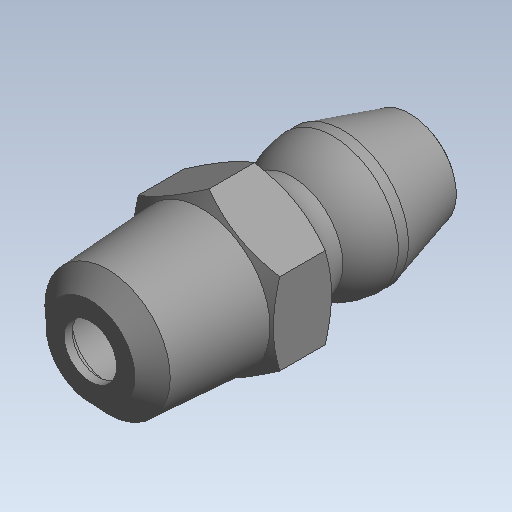
# Autodesk Inventor part: 1/4-28 SAE-LT
Saved by Autodesk Inventor 2020 (Build 240168000, 168)
## iProperties
Part Number: 1/4-28 SAE-LT
Material: Generic
Catalog Web Link: www.cadenas.de
Description: 1/4-28 SAE-LT-Grease Nipple
Vendor: SKF
Document SubType Name: Modeling
Designer: partserver
Manufacturer: SKF
Mass: 0.360827 g
Surface Area: 5.48785 cm^2
Volume: 0.360827 cm^3
Density: 1 g/cm^3
Appearance: PSOLRGB-175-175-175
Category: PARTsolutions
Company: SKF
PSOL_IDENT_0: {$CADENAS_DATA\23d-libs\skf\bearings_units_and_housings\bearing_units\ball_bearing_units\y-unit_acce
PSOL_IDENT_1: ssories\grease_nipple.prj},173 {VTYP=3D},{NB=1/4-28 SAE-LT},{LINA=1/4-28 SAE-LT},{NN=1/4-28 SAE-LT},
PSOL_IDENT_2: {DATE=20.08.2020 13:45:09},{GEOMDATE=29.07.2020 11:16:44},{VERSION=},{LINEID=10},{WBVAR=},{WBNUMERIC=
PSOL_IDENT_3: }  {NB=1/4-28 SAE-LT},{LINA=1/4-28 SAE-LT},{KT=DUMMY},{PN=1/4-28 SAE-LT}
NB: 1/4-28 SAE-LT
NN: 1/4-28 SAE-LT
NT: Grease Nipple
NBSYN: $PN.
LINA: 1/4-28 SAE-LT
CATALOG: SKF
PN: 1/4-28 SAE-LT
SUPPLIER: SKF
ARTICLENO: 1/4-28 SAE-LT
BOMINFO: 1/4-28 SAE-LT
CREATOR: CADENAS GmbH
Title: 1/4-28 SAE-LT
Author: Cadenas PARTsolutions
Comments: Grease Nipple
Autodesk Inventor part; units mm, degrees
ref_plane "YZ Plane" through (0, 0, 0) normal (1, 0, 0) x (0, 1, 0)
ref_plane "XZ Plane" through (0, 0, 0) normal (0, 1, 0) x (-1, 0, 0)
ref_plane "XY Plane" through (0, 0, 0) normal (0, 0, 1) x (1, 0, 0)
sketch "Sketch_1" plane through (0, 0, 0) normal (0, 0, 1) x (1, 0, 0)
  line L0 (0, -5.5) -> (0, 10.5)
  arc A0 (1, 10.2583) -> (0, 10.9) centre (0, 9.8) ccw
  line L1 (1, 10.2583) -> (1, 10.5)
  line L2 (1, 10.5) -> (2.0574, 10.5)
  line L3 (2.0574, 10.5) -> (2.3025, 10.3151)
  line L4 (2.3025, 10.3151) -> (3.25, 7)
  line L5 (3.25, 7) -> (3.25, 6.5)
  arc A1 (2.5, 4.5) -> (3.25, 6.5) centre (0.0009, 6.5778) ccw
  arc A2 (2.5, 4.5) -> (3.3937, 3) centre (5.3226, 5.1655) ccw
  line L6 (3.3937, 3) -> (5.5, 1.7839)
  line L7 (5.5, 1.7839) -> (5.5, 1.2161)
  line L8 (5.5, 1.2161) -> (3.3937, 0)
  line L9 (3.3937, 0) -> (3.1027, -4.6517)
  line L10 (3.1027, -4.6517) -> (2.1996, -5.5)
  line L11 (2.1996, -5.5) -> (1.3, -5.5)
  line L12 (1.3, -5.5) -> (1.3, -5.1)
  arc A3 (1.3, -5.1) -> (1.7, -4.7) centre (1.3, -4.7) ccw
  line L13 (1.7, -4.7) -> (1.7, 9.55)
  line L14 (1.7, 9.55) -> (1.0067, 10.2433)
  arc A4 (0, 8.7) -> (1.0067, 10.2433) centre (0, 9.8) ccw
  line L15 (0, 8.7) -> (0, 10.9)
  constraints: 32 end point, 10 point on circle, 5 centre point
revolve "Revolution1" add sketch "Sketch_1" angle 360 about axis through (0, -5.5, 0) along (0, -1, 0)
sketch "Sketch_2" plane through (0, 0, 0) normal (0, 1, 0) x (-1, 0, 0)
  line L0 (6, -6) -> (6, 6)
  line L1 (6, 6) -> (-6, 6)
  line L2 (-6, 6) -> (-6, -6)
  line L3 (-6, -6) -> (6, -6)
  line L4 (3.5, 2.0207) -> (0, 4.0415)
  line L5 (0, 4.0415) -> (-3.5, 2.0207)
  line L6 (-3.5, 2.0207) -> (-3.5, -2.0207)
  line L7 (-3.5, -2.0207) -> (0, -4.0415)
  line L8 (0, -4.0415) -> (3.5, -2.0207)
  line L9 (3.5, -2.0207) -> (3.5, 2.0207)
  constraints: 20 end point
extrude "Extrusion1" cut sketch "Sketch_2" along normal blind 3
ref_plane "gn_XY" through (0, 0, 0) normal (0, 0, 1) x (1, 0, 0)
ref_plane "gn_YZ" through (0, 0, 0) normal (1, 0, 0) x (0, 1, 0)
ref_plane "gn_ZX" through (0, 0, 0) normal (0, 1, 0) x (0, 0, 1)
body "Solid1"
